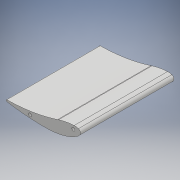
# Autodesk Inventor part: subflap
Saved by Autodesk Inventor 2018.3 (Build 223284000, 284)
## iProperties
Created: 2018-06-13
Part Number: subflap
Material: 一般
Document SubType Name: Modeling
Designer: ku_sk
Density: 1 g/cm^3
Appearance: 既定
Author: ku_sk
Autodesk Inventor part; units mm, degrees
ref_plane "YZ Plane" through (0, 0, 0) normal (1, 0, 0) x (0, 1, 0)
ref_plane "XZ Plane" through (0, 0, 0) normal (0, 1, 0) x (-1, 0, 0)
ref_plane "XY Plane" through (0, 0, 0) normal (0, 0, 1) x (1, 0, 0)
sketch "スケッチ1" plane through (0, 0, 0) normal (0, 1, 0) x (-1, 0, 0)
  circle A0 centre (8.3156, -0.3779) radius 3 projected
  circle A1 centre (94.4018, -18.6304) radius 3 projected
  arc A2 (74.4114, -25.2721) -> (141.066, -18.9974) centre (66.3691, 417.3255) ccw projected
  arc A3 (55.532, -25.0563) -> (74.4114, -25.2721) centre (68.6162, 293.6608) ccw projected
  arc A4 (20.857, -18.8926) -> (55.532, -25.0563) centre (60.903, 105.7764) ccw projected
  arc A5 (0.8403, -9.061) -> (20.857, -18.8926) centre (44.337, 54.204) ccw projected
  arc A6 (-4.8421, -3.5431) -> (0.8403, -9.061) centre (14.2278, 10.4108) ccw projected
  arc A7 (-1.8311, 5.7137) -> (-4.8421, -3.5431) centre (0, 0) ccw projected
  arc A8 (6.6893, 6.829) -> (-1.8311, 5.7137) centre (5.4934, -17.1412) ccw projected
  arc A9 (37.8866, 1.074) -> (6.6893, 6.829) centre (0.71, -113.022) ccw projected
  arc A10 (37.8866, 1.074) -> (39.7882, 0.4588) centre (186.5928, 457.4581) ccw projected
  arc A11 (39.7882, 0.4588) -> (140.8099, -15.8204) centre (143.7748, 324.1667) ccw projected
  arc A12 (141.066, -18.9974) -> (140.8099, -15.8204) centre (140.796, -17.4203) ccw projected
  point P0 (0, 0)
extrude "押し出し1" add sketch "スケッチ1" along normal mid plane 186
